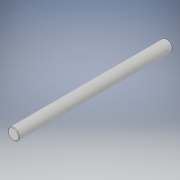
# Autodesk Inventor part: post
Saved by Autodesk Inventor 2017 (Build 210142000, 142)
## iProperties
Created: 2016-07-21
Part Number: post
Material: Generic
Document SubType Name: Modeling
Designer: Darien Morrow
Density: 1 g/cm^3
Appearance: Default
Author: Darien Morrow
Autodesk Inventor part; units mm, degrees
ref_plane "YZ Plane" through (0, 0, 0) normal (1, 0, 0) x (0, 1, 0)
ref_plane "XZ Plane" through (0, 0, 0) normal (0, 1, 0) x (-1, 0, 0)
ref_plane "XY Plane" through (0, 0, 0) normal (0, 0, 1) x (1, 0, 0)
sketch "Sketch1" plane through (0, 0, 0) normal (0, 0, 1) x (1, 0, 0)
  circle A0 centre (0, 0) radius 4.7625
  dimension "d0" = 9.525
  constraints: 2 coincident, 1 centre point
  measures "d0" diameter of A0
extrude "Extrusion1" add sketch "Sketch1" along normal blind 128.5875
sketch "Sketch2" plane through (0, 0, 0) normal (0, 0, -1) x (-1, 0, 0)
  point P0 (0, 0)
  point P1 (0, 0)
  constraints: 1 coincident
hole "Hole1" at (0, 0, 0) direction (0, 0, 1) diameter 3.302 depth 12.2936 tip angle 118 thread size "8-32 UNC" class "2B" standard "ANSI Unified Screw Threads"
chamfer "Chamfer1" distance 0.508 angle 45 1 edges at (-4.7625, 0, 128.5875)
body "Solid1"
